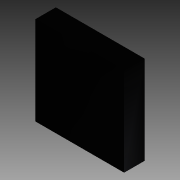
# Autodesk Inventor part: QFN16_4mmx4mm
Saved by Autodesk Inventor 2014 (Build 180170000, 170)
## iProperties
Created: 2014-11-22
Part Number: QFN16_4mmx4mm
Material: Phenolic Resin
Document SubType Name: Modeling
Designer: DV
Mass: 0.0210352 g
Surface Area: 0.493398 cm^2
Volume: 0.0152429 cm^3
Density: 1.38 g/cm^3
Appearance: Smooth - Light Orange
Author: DV
Autodesk Inventor part; units mm, degrees
ref_plane "YZ Plane" through (0, 0, 0) normal (1, 0, 0) x (0, 1, 0)
ref_plane "XZ Plane" through (0, 0, 0) normal (0, 1, 0) x (-1, 0, 0)
ref_plane "XY Plane" through (0, 0, 0) normal (0, 0, 1) x (1, 0, 0)
sketch "Sketch1" plane through (0, 0, 0) normal (0, 0, 1) x (1, 0, 0)
  line L0 (-2, 2) -> (2, 2)
  line L1 (2, 2) -> (2, -2)
  line L2 (2, -2) -> (-2, -2)
  line L3 (-2, -2) -> (-2, 2)
  point P0 (0, 0)
  dimension "d0" = 4
  dimension "d1" = 4
  dimension "d22" = 2
  dimension "d23" = 2
  constraints: 8 end point, 2 parallel, 1 horizontal, 1 perpendicular
  measures "d0" distance of L1.end L2.end
  measures "d1" distance of L2.end L0.start
  measures "d22" distance from line of point (0, 0) L3
  measures "d23" distance from line of point (0, 0) L2
extrude "Extrusion1" add sketch "Sketch1" along normal blind 0.92
ref_plane "Work Plane1" through (0, 0, 1) normal (0, 0, 1) x (1, 0, 0)
sketch "Sketch2" plane through (0, 0, 1) normal (0, 0, 1) x (1, 0, 0)
  line L0 (2, 2) -> (-2, 2) projected
  line L1 (-2, 2) -> (-2, -2) projected
  line L2 (-2, -2) -> (2, -2) projected
  line L3 (2, -2) -> (2, 2) projected
  line L4 (-1.125, -2) -> (-1.125, -1.6163)
  line L5 (-0.825, -1.6163) -> (-0.825, -2)
  arc A0 (-0.825, -1.6163) -> (-1.125, -1.6163) centre (-0.975, -1.6163) ccw
  line L6 (-0.475, -2) -> (-0.475, -1.6163)
  line L7 (-0.175, -1.6163) -> (-0.175, -2)
  arc A1 (-0.175, -1.6163) -> (-0.475, -1.6163) centre (-0.325, -1.6163) ccw
  line L8 (0.175, -2) -> (0.175, -1.6163)
  line L9 (0.475, -1.6163) -> (0.475, -2)
  arc A2 (0.475, -1.6163) -> (0.175, -1.6163) centre (0.325, -1.6163) ccw
  line L10 (0.825, -2) -> (0.825, -1.6163)
  line L11 (1.125, -1.6163) -> (1.125, -2)
  arc A3 (1.125, -1.6163) -> (0.825, -1.6163) centre (0.975, -1.6163) ccw
  line L12 (0, 0) -> (0, -2.7079) construction
  dimension "d7" = 0.3837
  dimension "d8" = 0.3
  dimension "d11" = 0.65
  dimension "d16" = 0.325
  constraints: 18 end point, 8 point on circle, 4 centre point, 2 parallel, 2 point on line, 1 horizontal, 1 perpendicular, 24 other
  measures "d7" distance from line of L2 A0.centre
  measures "d8" distance between parallel lines of L5 L4
  measures "d11" distance of A0.centre A1.centre
  measures "d16" distance from line of A1.centre L12
extrude "Extrusion2" add sketch "Sketch2" against normal blind 0.2 contours L4 A0 L5 L2
pattern_linear "Rectangular Pattern1" count 4 spacing 0.65 along (1, 0, 0) of "Extrusion2"
pattern_circular "Circular Pattern1" count 4 over 360 about axis through (0, 0, -10) along (0, 0, 1) of "Extrusion2", "Rectangular Pattern1"
sketch "Sketch3" plane through (0, 0, 1) normal (0, 0, 1) x (1, 0, 0)
  line L0 (-1.016, 1.016) -> (1.016, 1.016)
  line L1 (1.016, 1.016) -> (1.016, -1.016)
  line L2 (1.016, -1.016) -> (-1.016, -1.016)
  line L3 (-1.016, -1.016) -> (-1.016, 1.016)
  point P0 (0, 0)
  dimension "d27" = 2.032
  dimension "d28" = 2.032
  dimension "d29" = 1.016
  dimension "d30" = 1.016
  constraints: 8 end point, 2 parallel, 1 horizontal, 1 perpendicular
  measures "d27" distance of L1.end L2.end
  measures "d28" distance of L0.end L1.end
  measures "d29" distance from line of L1 point (0, 0)
  measures "d30" distance from line of L2 point (0, 0)
extrude "Extrusion3" add sketch "Sketch3" against normal blind 0.2
equation "\"d22\" = 0.5 * d0"
equation "\"d23\" = 0.5 * d1"
equation "\"d29\" = 0.5 * d27"
equation "\"d30\" = 0.5 * d28"
body "Solid1"
